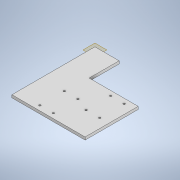
# Autodesk Inventor part: borard2_L
Saved by Autodesk Inventor 2020 (Build 240168000, 168)
## iProperties
Created: 2022-07-25
Part Number: borard2_L
Material: 일반
Document SubType Name: Modeling
Designer: SeungJin
Density: 1 g/cm^3
Appearance: 기본값
Author: SeungJin
Autodesk Inventor part; units mm, degrees
ref_plane "YZ Plane" through (0, 0, 0) normal (1, 0, 0) x (0, 1, 0)
ref_plane "XZ Plane" through (0, 0, 0) normal (0, 1, 0) x (-1, 0, 0)
ref_plane "XY Plane" through (0, 0, 0) normal (0, 0, 1) x (1, 0, 0)
ref_plane "작업 평면1" through (-145.5, 0, 75) normal (0, 1, 0) x (1, 0, 0)
sketch "스케치1" plane through (-145.5, 0, 75) normal (0, 1, 0) x (1, 0, 0)
  line L0 (0, -152.5) -> (185.5, -152.5)
  line L1 (185.5, -152.5) -> (185.5, 10)
  line L2 (185.5, 10) -> (75, 10)
  line L3 (75, 10) -> (75, 0)
  line L4 (75, 0) -> (0, 0)
  line L5 (0, 0) -> (0, -152.5)
  line L6 (185.5, 10) -> (75, 10)
  line L7 (185.5, 10) -> (34.5, 10)
  line L8 (34.5, 10) -> (34.5, -55)
  line L9 (34.5, -55) -> (185.5, -55)
  line L10 (185.5, -55) -> (185.5, 10)
  line L11 (44.5, -55) -> (44.5, 10)
  line L12 (195.5, 10) -> (195.5, -55)
  line L13 (134.5, -152.5) -> (134.5, -55)
  point P0 (44.5, 0)
  dimension "d1" = 151
  dimension "d2" = 65
  dimension "d3" = 10
  dimension "d4" = 10
  dimension "d27" = 90
  constraints: 28 end point, 4 point on line, 1 perpendicular, 1 other
  measures "d1" distance of L9.end L8.end
  measures "d2" distance of L8.end L7.end
  measures "d3" distance between parallel lines of L11 L8
  measures "d4" distance between parallel lines of L12 L1
  measures "d27" distance between parallel lines of L13 L11
extrude "돌출1" add sketch "스케치1" along normal blind 5 contours L5 L4 L8 L9 L13 L0 | L4 L11 L9 L8
sketch "스케치3" plane through (-145.5, 0, 75) normal (0, -1, 0) x (1, 0, 0)
  line L0 (44.5, 55) -> (44.5, 0) projected
  line L1 (134.5, 55) -> (44.5, 55) projected
  line L2 (0, 152.5) -> (134.5, 152.5) projected
  line L3 (0, 0) -> (0, 152.5) projected
  line L4 (44.5, 0) -> (0, 0) projected
  line L5 (44.5, 0) -> (0, 0) projected
  line L6 (134.5, 152.5) -> (134.5, 55) projected
  line L7 (30, 146.25) -> (80, 146.25)
  line L8 (80, 146.25) -> (80, 96.25)
  line L9 (80, 96.25) -> (30, 96.25)
  line L10 (30, 96.25) -> (30, 146.25)
  line L11 (130, 61.25) -> (80, 61.25)
  line L12 (80, 61.25) -> (80, 111.25)
  line L13 (80, 111.25) -> (130, 111.25)
  line L14 (130, 111.25) -> (130, 61.25)
  line L15 (42.5, 143.75) -> (67.5, 143.75)
  line L16 (67.5, 143.75) -> (67.5, 98.75)
  line L17 (67.5, 98.75) -> (42.5, 98.75)
  line L18 (42.5, 98.75) -> (42.5, 143.75)
  line L19 (92.5, 108.75) -> (117.5, 108.75)
  line L20 (117.5, 108.75) -> (117.5, 63.75)
  line L21 (117.5, 63.75) -> (92.5, 63.75)
  line L22 (92.5, 63.75) -> (92.5, 108.75)
  point P0 (145.5, -75)
  point P1 (130, 103.75)
  point P2 (134.5, 103.75)
  point P3 (42.5, 121.25)
  point P4 (30, 121.25)
  point P5 (92.5, 86.25)
  point P6 (80, 86.25)
  point P7 (105, 108.75)
  point P8 (105, 111.25)
  point P9 (55, 143.75)
  point P10 (55, 146.25)
  dimension "d32" = 50
  dimension "d34" = 50
  dimension "d35" = 25
  dimension "d36" = 45
  dimension "d37" = 25
  dimension "d38" = 45
  dimension "d39" = 50
  dimension "d40" = 50
  constraints: 32 end point, 9 midpoint, 8 coincident, 8 parallel, 4 horizontal, 4 perpendicular, 3 horizontal alignment, 2 vertical alignment, 1 point on line, 2 other
  measures "d32" distance of L8.end L9.end
  measures "d34" distance of L11.end L12.end
  measures "d35" distance of L16.end L17.end
  measures "d36" distance of L15.end L16.end
  measures "d37" distance of L20.end L21.end
  measures "d38" distance of L19.end L20.end
  measures "d39" distance between parallel lines of L9 L7
  measures "d40" distance between parallel lines of L12 L14
hole "구멍1" at (-103, 0, 218.75) at (-103, 0, 173.75) at (-78, 0, 218.75) at (-78, 0, 173.75) at (-53, 0, 183.75) at (-28, 0, 183.75) at (-28, 0, 138.75) at (-53, 0, 138.75) direction (0, 1, 0) diameter 3.4 end through all counterbore diameter 6 counterbore depth 3 clearance for "Hex Head Cap Screw ISO 24017" size "M3" standard "ISO"
